Autodesk Fusion 360 part; units mm, degrees
(part 2 of 4)
  arc A294 (-148.6977, 144.525) -> (-148.6977, 141.525) centre (-148.6977, 143.025) ccw
  arc A295 (-138.6977, 141.525) -> (-138.6977, 144.525) centre (-138.6977, 143.025) ccw
  line L447 (-148.6977, 144.525) -> (-138.6977, 144.525)
  line L448 (-148.6977, 141.525) -> (-143.6977, 141.525)
  line L449 (-138.6977, 141.525) -> (-143.6977, 141.525)
  arc A296 (-128.6977, 144.525) -> (-128.6977, 141.525) centre (-128.6977, 143.025) ccw
  arc A297 (-118.6977, 141.525) -> (-118.6977, 144.525) centre (-118.6977, 143.025) ccw
  line L450 (-128.6977, 144.525) -> (-118.6977, 144.525)
  line L451 (-128.6977, 141.525) -> (-123.6977, 141.525)
  line L452 (-118.6977, 141.525) -> (-123.6977, 141.525)
  arc A298 (-228.6977, 154.525) -> (-228.6977, 151.525) centre (-228.6977, 153.025) ccw
  arc A299 (-218.6977, 151.525) -> (-218.6977, 154.525) centre (-218.6977, 153.025) ccw
  line L453 (-228.6977, 154.525) -> (-218.6977, 154.525)
  line L454 (-228.6977, 151.525) -> (-223.6977, 151.525)
  line L455 (-218.6977, 151.525) -> (-223.6977, 151.525)
  arc A300 (-208.6977, 154.525) -> (-208.6977, 151.525) centre (-208.6977, 153.025) ccw
  arc A301 (-198.6977, 151.525) -> (-198.6977, 154.525) centre (-198.6977, 153.025) ccw
  line L456 (-208.6977, 154.525) -> (-198.6977, 154.525)
  line L457 (-208.6977, 151.525) -> (-203.6977, 151.525)
  line L458 (-198.6977, 151.525) -> (-203.6977, 151.525)
  arc A302 (-188.6977, 154.525) -> (-188.6977, 151.525) centre (-188.6977, 153.025) ccw
  arc A303 (-178.6977, 151.525) -> (-178.6977, 154.525) centre (-178.6977, 153.025) ccw
  line L459 (-188.6977, 154.525) -> (-178.6977, 154.525)
  line L460 (-188.6977, 151.525) -> (-183.6977, 151.525)
  line L461 (-178.6977, 151.525) -> (-183.6977, 151.525)
  arc A304 (-168.6977, 154.525) -> (-168.6977, 151.525) centre (-168.6977, 153.025) ccw
  arc A305 (-158.6977, 151.525) -> (-158.6977, 154.525) centre (-158.6977, 153.025) ccw
  line L462 (-168.6977, 154.525) -> (-158.6977, 154.525)
  line L463 (-168.6977, 151.525) -> (-163.6977, 151.525)
  line L464 (-158.6977, 151.525) -> (-163.6977, 151.525)
  arc A306 (-148.6977, 154.525) -> (-148.6977, 151.525) centre (-148.6977, 153.025) ccw
  arc A307 (-138.6977, 151.525) -> (-138.6977, 154.525) centre (-138.6977, 153.025) ccw
  line L465 (-148.6977, 154.525) -> (-138.6977, 154.525)
  line L466 (-148.6977, 151.525) -> (-143.6977, 151.525)
  line L467 (-138.6977, 151.525) -> (-143.6977, 151.525)
  arc A308 (-128.6977, 154.525) -> (-128.6977, 151.525) centre (-128.6977, 153.025) ccw
  arc A309 (-118.6977, 151.525) -> (-118.6977, 154.525) centre (-118.6977, 153.025) ccw
  line L468 (-128.6977, 154.525) -> (-118.6977, 154.525)
  line L469 (-128.6977, 151.525) -> (-123.6977, 151.525)
  line L470 (-118.6977, 151.525) -> (-123.6977, 151.525)
  arc A310 (-228.6977, 164.525) -> (-228.6977, 161.525) centre (-228.6977, 163.025) ccw
  arc A311 (-218.6977, 161.525) -> (-218.6977, 164.525) centre (-218.6977, 163.025) ccw
  line L471 (-228.6977, 164.525) -> (-218.6977, 164.525)
  line L472 (-228.6977, 161.525) -> (-223.6977, 161.525)
  line L473 (-218.6977, 161.525) -> (-223.6977, 161.525)
  arc A312 (-208.6977, 164.525) -> (-208.6977, 161.525) centre (-208.6977, 163.025) ccw
  arc A313 (-198.6977, 161.525) -> (-198.6977, 164.525) centre (-198.6977, 163.025) ccw
  line L474 (-208.6977, 164.525) -> (-198.6977, 164.525)
  line L475 (-208.6977, 161.525) -> (-203.6977, 161.525)
  line L476 (-198.6977, 161.525) -> (-203.6977, 161.525)
  arc A314 (-188.6977, 164.525) -> (-188.6977, 161.525) centre (-188.6977, 163.025) ccw
  arc A315 (-178.6977, 161.525) -> (-178.6977, 164.525) centre (-178.6977, 163.025) ccw
  line L477 (-188.6977, 164.525) -> (-178.6977, 164.525)
  line L478 (-188.6977, 161.525) -> (-183.6977, 161.525)
  line L479 (-178.6977, 161.525) -> (-183.6977, 161.525)
  arc A316 (-168.6977, 164.525) -> (-168.6977, 161.525) centre (-168.6977, 163.025) ccw
  arc A317 (-158.6977, 161.525) -> (-158.6977, 164.525) centre (-158.6977, 163.025) ccw
  line L480 (-168.6977, 164.525) -> (-158.6977, 164.525)
  line L481 (-168.6977, 161.525) -> (-163.6977, 161.525)
  line L482 (-158.6977, 161.525) -> (-163.6977, 161.525)
  arc A318 (-148.6977, 164.525) -> (-148.6977, 161.525) centre (-148.6977, 163.025) ccw
  arc A319 (-138.6977, 161.525) -> (-138.6977, 164.525) centre (-138.6977, 163.025) ccw
  line L483 (-148.6977, 164.525) -> (-138.6977, 164.525)
  line L484 (-148.6977, 161.525) -> (-143.6977, 161.525)
  line L485 (-138.6977, 161.525) -> (-143.6977, 161.525)
  arc A320 (-208.6977, 174.525) -> (-208.6977, 171.525) centre (-208.6977, 173.025) ccw
  arc A321 (-198.6977, 171.525) -> (-198.6977, 174.525) centre (-198.6977, 173.025) ccw
  line L486 (-208.6977, 174.525) -> (-198.6977, 174.525)
  line L487 (-208.6977, 171.525) -> (-203.6977, 171.525)
  line L488 (-198.6977, 171.525) -> (-203.6977, 171.525)
  arc A322 (-188.6977, 174.525) -> (-188.6977, 171.525) centre (-188.6977, 173.025) ccw
  arc A323 (-178.6977, 171.525) -> (-178.6977, 174.525) centre (-178.6977, 173.025) ccw
  line L489 (-188.6977, 174.525) -> (-178.6977, 174.525)
  line L490 (-188.6977, 171.525) -> (-183.6977, 171.525)
  line L491 (-178.6977, 171.525) -> (-183.6977, 171.525)
  arc A324 (-168.6977, 174.525) -> (-168.6977, 171.525) centre (-168.6977, 173.025) ccw
  arc A325 (-158.6977, 171.525) -> (-158.6977, 174.525) centre (-158.6977, 173.025) ccw
  line L492 (-168.6977, 174.525) -> (-158.6977, 174.525)
  line L493 (-168.6977, 171.525) -> (-163.6977, 171.525)
  line L494 (-158.6977, 171.525) -> (-163.6977, 171.525)
  arc A326 (-148.6977, 174.525) -> (-148.6977, 171.525) centre (-148.6977, 173.025) ccw
  arc A327 (-138.6977, 171.525) -> (-138.6977, 174.525) centre (-138.6977, 173.025) ccw
  line L495 (-148.6977, 174.525) -> (-138.6977, 174.525)
  line L496 (-148.6977, 171.525) -> (-143.6977, 171.525)
  line L497 (-138.6977, 171.525) -> (-143.6977, 171.525)
  arc A328 (-208.6977, 184.525) -> (-208.6977, 181.525) centre (-208.6977, 183.025) ccw
  arc A329 (-198.6977, 181.525) -> (-198.6977, 184.525) centre (-198.6977, 183.025) ccw
  line L498 (-208.6977, 184.525) -> (-198.6977, 184.525)
  line L499 (-208.6977, 181.525) -> (-203.6977, 181.525)
  line L500 (-198.6977, 181.525) -> (-203.6977, 181.525)
  arc A330 (-188.6977, 184.525) -> (-188.6977, 181.525) centre (-188.6977, 183.025) ccw
  arc A331 (-178.6977, 181.525) -> (-178.6977, 184.525) centre (-178.6977, 183.025) ccw
  line L501 (-188.6977, 184.525) -> (-178.6977, 184.525)
  line L502 (-188.6977, 181.525) -> (-183.6977, 181.525)
  line L503 (-178.6977, 181.525) -> (-183.6977, 181.525)
  arc A332 (-168.6977, 184.525) -> (-168.6977, 181.525) centre (-168.6977, 183.025) ccw
  arc A333 (-158.6977, 181.525) -> (-158.6977, 184.525) centre (-158.6977, 183.025) ccw
  line L504 (-168.6977, 184.525) -> (-158.6977, 184.525)
  line L505 (-168.6977, 181.525) -> (-163.6977, 181.525)
  line L506 (-158.6977, 181.525) -> (-163.6977, 181.525)
  arc A334 (-148.6977, 184.525) -> (-148.6977, 181.525) centre (-148.6977, 183.025) ccw
  arc A335 (-138.6977, 181.525) -> (-138.6977, 184.525) centre (-138.6977, 183.025) ccw
  line L507 (-148.6977, 184.525) -> (-138.6977, 184.525)
  line L508 (-148.6977, 181.525) -> (-143.6977, 181.525)
  line L509 (-138.6977, 181.525) -> (-143.6977, 181.525)
  line L510 (-269.4662, 146.0492) -> (-250, 146.0218)
  line L511 (-269.5337, 0.009) -> (-249.9865, 0)
  line L512 (-105.9194, 0) -> (-90, 0)
  line L513 (-90, 0) -> (-60, 38.025)
  line L514 (-60, 38.025) -> (-17.3954, 46.901)
  line L515 (-17.3954, 99.149) -> (-17.3954, 46.901)
  line L516 (-60, 108.025) -> (-17.3954, 99.149)
  line L517 (-90, 146.05) -> (-60, 108.025)
  line L518 (-105.9194, 146.05) -> (-90, 146.05)
  line L519 (-269.4662, 146.0492) -> (-269.5337, 0.009)
  line L520 (-46.3999, 83.0262) -> (-53.3999, 83.0262)
  line L521 (-53.3999, 83.0262) -> (-53.3999, 63.0262)
  line L522 (-53.3999, 63.0262) -> (-46.3999, 63.0262)
  line L523 (-46.3999, 63.0262) -> (-46.3999, 83.0262)
  line L524 (-46.3999, 83.0262) -> (-53.3999, 63.0262) construction
  line L525 (-53.3999, 83.0262) -> (-46.3999, 63.0262) construction
  point P0 (-143.6977, 73.025)
  point P1 (-203.6977, -36.975)
  point P2 (-183.6977, -36.975)
  point P3 (-163.6977, -36.975)
  point P4 (-143.6977, -36.975)
  point P5 (-203.6977, -26.975)
  point P6 (-183.6977, -26.975)
  point P7 (-163.6977, -26.975)
  point P8 (-143.6977, -26.975)
  point P9 (-223.6977, -16.975)
  point P10 (-203.6977, -16.975)
  point P11 (-183.6977, -16.975)
  point P12 (-163.6977, -16.975)
  point P13 (-143.6977, -16.975)
  point P14 (-223.6977, -6.975)
  point P15 (-203.6977, -6.975)
  point P16 (-183.6977, -6.975)
  point P17 (-163.6977, -6.975)
  point P18 (-143.6977, -6.975)
  point P19 (-123.6977, -6.975)
  point P20 (-223.6977, 3.025)
  point P21 (-203.6977, 3.025)
  point P22 (-183.6977, 3.025)
  point P23 (-163.6977, 3.025)
  point P24 (-143.6977, 3.025)
  point P25 (-123.6977, 3.025)
  point P26 (-243.6977, 13.025)
  point P27 (-223.6977, 13.025)
  point P28 (-203.6977, 13.025)
  point P29 (-183.6977, 13.025)
  point P30 (-163.6977, 13.025)
  point P31 (-143.6977, 13.025)
  point P32 (-123.6977, 13.025)
  point P33 (-103.6977, 13.025)
  point P34 (-243.6977, 23.025)
  point P35 (-223.6977, 23.025)
  point P36 (-203.6977, 23.025)
  point P37 (-183.6977, 23.025)
  point P38 (-163.6977, 23.025)
  point P39 (-143.6977, 23.025)
  point P40 (-123.6977, 23.025)
  point P41 (-103.6977, 23.025)
  point P42 (-243.6977, 33.025)
  point P43 (-223.6977, 33.025)
  point P44 (-203.6977, 33.025)
  point P45 (-183.6977, 33.025)
  point P46 (-163.6977, 33.025)
  point P47 (-143.6977, 33.025)
  point P48 (-123.6977, 33.025)
  point P49 (-103.6977, 33.025)
  point P50 (-83.6977, 33.025)
  point P51 (-243.6977, 43.025)
  point P52 (-223.6977, 43.025)
  point P53 (-203.6977, 43.025)
  point P54 (-183.6977, 43.025)
  point P55 (-163.6977, 43.025)
  point P56 (-143.6977, 43.025)
  point P57 (-123.6977, 43.025)
  point P58 (-103.6977, 43.025)
  point P59 (-83.6977, 43.025)
  point P60 (-63.6977, 43.025)
  point P61 (-43.6977, 43.025)
  point P62 (-243.6977, 53.025)
  point P63 (-223.6977, 53.025)
  point P64 (-203.6977, 53.025)
  point P65 (-183.6977, 53.025)
  point P66 (-163.6977, 53.025)
  point P67 (-143.6977, 53.025)
  point P68 (-123.6977, 53.025)
  point P69 (-103.6977, 53.025)
  point P70 (-83.6977, 53.025)
  point P71 (-63.6977, 53.025)
  point P72 (-243.6977, 63.025)
  point P73 (-223.6977, 63.025)
  point P74 (-203.6977, 63.025)
  point P75 (-183.6977, 63.025)
  point P76 (-163.6977, 63.025)
  point P77 (-143.6977, 63.025)
  point P78 (-123.6977, 63.025)
  point P79 (-103.6977, 63.025)
  point P80 (-83.6977, 63.025)
  point P81 (-63.6977, 63.025)
  point P82 (-243.6977, 73.025)
  point P83 (-223.6977, 73.025)
  point P84 (-203.6977, 73.025)
  point P85 (-183.6977, 73.025)
  point P86 (-163.6977, 73.025)
  point P87 (-123.6977, 73.025)
  point P88 (-103.6977, 73.025)
  point P89 (-83.6977, 73.025)
  point P90 (-63.6977, 73.025)
  point P91 (-243.6977, 83.025)
  point P92 (-223.6977, 83.025)
  point P93 (-203.6977, 83.025)
  point P94 (-183.6977, 83.025)
  point P95 (-163.6977, 83.025)
  point P96 (-143.6977, 83.025)
  point P97 (-123.6977, 83.025)
  point P98 (-103.6977, 83.025)
  point P99 (-83.6977, 83.025)
  point P100 (-63.6977, 83.025)
  point P101 (-243.6977, 93.025)
  point P102 (-223.6977, 93.025)
  point P103 (-203.6977, 93.025)
  point P104 (-183.6977, 93.025)
  point P105 (-163.6977, 93.025)
  point P106 (-143.6977, 93.025)
  point P107 (-123.6977, 93.025)
  point P108 (-103.6977, 93.025)
  point P109 (-83.6977, 93.025)
  point P110 (-63.6977, 93.025)
  point P111 (-243.6977, 103.025)
  point P112 (-223.6977, 103.025)
  point P113 (-203.6977, 103.025)
  point P114 (-183.6977, 103.025)
  point P115 (-163.6977, 103.025)
  point P116 (-143.6977, 103.025)
  point P117 (-123.6977, 103.025)
  point P118 (-103.6977, 103.025)
  point P119 (-83.6977, 103.025)
  point P120 (-243.6977, 113.025)
  point P121 (-223.6977, 113.025)
  point P122 (-203.6977, 113.025)
  point P123 (-183.6977, 113.025)
  point P124 (-163.6977, 113.025)
  point P125 (-143.6977, 113.025)
  point P126 (-123.6977, 113.025)
  point P127 (-103.6977, 113.025)
  point P128 (-83.6977, 113.025)
  point P129 (-243.6977, 123.025)
  point P130 (-223.6977, 123.025)
  point P131 (-203.6977, 123.025)
  point P132 (-183.6977, 123.025)
  point P133 (-163.6977, 123.025)
  point P134 (-143.6977, 123.025)
  point P135 (-123.6977, 123.025)
  point P136 (-103.6977, 123.025)
  point P137 (-243.6977, 133.025)
  point P138 (-223.6977, 133.025)
  point P139 (-203.6977, 133.025)
  point P140 (-183.6977, 133.025)
  point P141 (-163.6977, 133.025)
  point P142 (-143.6977, 133.025)
  point P143 (-123.6977, 133.025)
  point P144 (-103.6977, 133.025)
  point P145 (-223.6977, 143.025)
  point P146 (-203.6977, 143.025)
  point P147 (-183.6977, 143.025)
  point P148 (-163.6977, 143.025)
  point P149 (-143.6977, 143.025)
  point P150 (-123.6977, 143.025)
  point P151 (-223.6977, 153.025)
  point P152 (-203.6977, 153.025)
  point P153 (-183.6977, 153.025)
  point P154 (-163.6977, 153.025)
  point P155 (-143.6977, 153.025)
  point P156 (-123.6977, 153.025)
  point P157 (-223.6977, 163.025)
  point P158 (-203.6977, 163.025)
  point P159 (-183.6977, 163.025)
  point P160 (-163.6977, 163.025)
  point P161 (-143.6977, 163.025)
  point P162 (-203.6977, 173.025)
  point P163 (-183.6977, 173.025)
  point P164 (-163.6977, 173.025)
  point P165 (-143.6977, 173.025)
  point P166 (-203.6977, 183.025)
  point P167 (-183.6977, 183.025)
  point P168 (-163.6977, 183.025)
  point P169 (-143.6977, 183.025)
  point P170 (-49.8999, 73.0262)
  dimension "d82" = 10
  dimension "d83" = 3
  dimension "d86" = 20
  dimension "d87" = 10
  dimension "d120" = 7
  dimension "d121" = 20
  dimension "d122" = 219.6
  constraint horizontal L6
  constraint parallel L6 L7
  constraint tangent A1 L8
  constraint horizontal L512
  constraint vertical L515
  constraint horizontal L518
  constraint perpendicular L511 L519
  constraint horizontal L520
  constraint perpendicular L520 L521
  constraint parallel L520 L522
  constraint parallel L521 L523
  constraint coincident L524 P170
  constraint coincident L525 P170
  measures "d82" distance of L7.start L7.end
  measures "d83" distance of A1.end L7.start
  measures "d120" distance of L521.end L522.end
  measures "d121" distance of L520.end L521.end
  measures "d122" distance of L519 P170
extrude "Extrude3" add sketch "Sketch2" along normal blind 5 makes body 1
sketch "Sketch8" plane through (0, 5, 0) normal (0, 1, 0) x (-1, 0, 0)
  arc A0 (248.6977, -94.525) -> (248.6977, -91.525) centre (248.6977, -93.025) ccw
  line L0 (248.6977, -94.525) -> (238.6977, -94.525)
  arc A1 (238.6977, -91.525) -> (238.6977, -94.525) centre (238.6977, -93.025) ccw
  line L1 (238.6977, -91.525) -> (248.6977, -91.525)
  arc A2 (208.6977, -154.525) -> (208.6977, -151.525) centre (208.6977, -153.025) ccw
  line L2 (208.6977, -154.525) -> (198.6977, -154.525)
  arc A3 (198.6977, -151.525) -> (198.6977, -154.525) centre (198.6977, -153.025) ccw
  line L3 (198.6977, -151.525) -> (208.6977, -151.525)
  arc A4 (168.6977, -64.525) -> (168.6977, -61.525) centre (168.6977, -63.025) ccw
  line L4 (168.6977, -64.525) -> (158.6977, -64.525)
  arc A5 (158.6977, -61.525) -> (158.6977, -64.525) centre (158.6977, -63.025) ccw
  line L5 (158.6977, -61.525) -> (168.6977, -61.525)
  arc A6 (228.6977, -114.525) -> (228.6977, -111.525) centre (228.6977, -113.025) ccw
  line L6 (228.6977, -114.525) -> (218.6977, -114.525)
  arc A7 (218.6977, -111.525) -> (218.6977, -114.525) centre (218.6977, -113.025) ccw
  line L7 (218.6977, -111.525) -> (228.6977, -111.525)
  arc A8 (128.6977, -154.525) -> (128.6977, -151.525) centre (128.6977, -153.025) ccw
  line L8 (128.6977, -154.525) -> (118.6977, -154.525)
  arc A9 (118.6977, -151.525) -> (118.6977, -154.525) centre (118.6977, -153.025) ccw
  line L9 (118.6977, -151.525) -> (128.6977, -151.525)
  arc A10 (228.6977, -144.525) -> (228.6977, -141.525) centre (228.6977, -143.025) ccw
  line L10 (228.6977, -144.525) -> (218.6977, -144.525)
  arc A11 (218.6977, -141.525) -> (218.6977, -144.525) centre (218.6977, -143.025) ccw
  line L11 (218.6977, -141.525) -> (228.6977, -141.525)
  arc A12 (168.6977, -144.525) -> (168.6977, -141.525) centre (168.6977, -143.025) ccw
  line L12 (168.6977, -144.525) -> (158.6977, -144.525)
  arc A13 (158.6977, -141.525) -> (158.6977, -144.525) centre (158.6977, -143.025) ccw
  line L13 (158.6977, -141.525) -> (168.6977, -141.525)
  arc A14 (168.6977, -154.525) -> (168.6977, -151.525) centre (168.6977, -153.025) ccw
  line L14 (168.6977, -154.525) -> (158.6977, -154.525)
  arc A15 (158.6977, -151.525) -> (158.6977, -154.525) centre (158.6977, -153.025) ccw
  line L15 (158.6977, -151.525) -> (168.6977, -151.525)
  arc A16 (248.6977, -74.525) -> (248.6977, -71.525) centre (248.6977, -73.025) ccw
  line L16 (248.6977, -74.525) -> (238.6977, -74.525)
  arc A17 (238.6977, -71.525) -> (238.6977, -74.525) centre (238.6977, -73.025) ccw
  line L17 (238.6977, -71.525) -> (248.6977, -71.525)
  arc A18 (248.6977, -114.525) -> (248.6977, -111.525) centre (248.6977, -113.025) ccw
  line L18 (248.6977, -114.525) -> (238.6977, -114.525)
  arc A19 (238.6977, -111.525) -> (238.6977, -114.525) centre (238.6977, -113.025) ccw
  line L19 (238.6977, -111.525) -> (248.6977, -111.525)
  arc A20 (148.6977, -174.525) -> (148.6977, -171.525) centre (148.6977, -173.025) ccw
  line L20 (148.6977, -174.525) -> (138.6977, -174.525)
  arc A21 (138.6977, -171.525) -> (138.6977, -174.525) centre (138.6977, -173.025) ccw
  line L21 (138.6977, -171.525) -> (148.6977, -171.525)
  arc A22 (128.6977, -134.525) -> (128.6977, -131.525) centre (128.6977, -133.025) ccw
  line L22 (128.6977, -134.525) -> (118.6977, -134.525)
  arc A23 (118.6977, -131.525) -> (118.6977, -134.525) centre (118.6977, -133.025) ccw
  line L23 (118.6977, -131.525) -> (128.6977, -131.525)
  arc A24 (128.6977, -144.525) -> (128.6977, -141.525) centre (128.6977, -143.025) ccw
  line L24 (128.6977, -144.525) -> (118.6977, -144.525)
  arc A25 (118.6977, -141.525) -> (118.6977, -144.525) centre (118.6977, -143.025) ccw
  line L25 (118.6977, -141.525) -> (128.6977, -141.525)
  arc A26 (88.6977, -84.525) -> (88.6977, -81.525) centre (88.6977, -83.025) ccw
  line L26 (88.6977, -84.525) -> (78.6977, -84.525)
  arc A27 (78.6977, -81.525) -> (78.6977, -84.525) centre (78.6977, -83.025) ccw
  line L27 (78.6977, -81.525) -> (88.6977, -81.525)
  arc A28 (228.6977, -74.525) -> (228.6977, -71.525) centre (228.6977, -73.025) ccw
  line L28 (228.6977, -74.525) -> (218.6977, -74.525)
  arc A29 (218.6977, -71.525) -> (218.6977, -74.525) centre (218.6977, -73.025) ccw
  line L29 (218.6977, -71.525) -> (228.6977, -71.525)
  arc A30 (108.6977, -104.525) -> (108.6977, -101.525) centre (108.6977, -103.025) ccw
  line L30 (108.6977, -104.525) -> (98.6977, -104.525)
  arc A31 (98.6977, -101.525) -> (98.6977, -104.525) centre (98.6977, -103.025) ccw
  line L31 (98.6977, -101.525) -> (108.6977, -101.525)
  arc A32 (108.6977, -134.525) -> (108.6977, -131.525) centre (108.6977, -133.025) ccw
  line L32 (108.6977, -134.525) -> (98.6977, -134.525)
  arc A33 (98.6977, -131.525) -> (98.6977, -134.525) centre (98.6977, -133.025) ccw
  line L33 (98.6977, -131.525) -> (108.6977, -131.525)
  arc A34 (148.6977, -134.525) -> (148.6977, -131.525) centre (148.6977, -133.025) ccw
  line L34 (148.6977, -134.525) -> (138.6977, -134.525)
  arc A35 (138.6977, -131.525) -> (138.6977, -134.525) centre (138.6977, -133.025) ccw
  line L35 (138.6977, -131.525) -> (148.6977, -131.525)
  arc A36 (168.6977, -184.525) -> (168.6977, -181.525) centre (168.6977, -183.025) ccw
  line L36 (168.6977, -184.525) -> (158.6977, -184.525)
  arc A37 (158.6977, -181.525) -> (158.6977, -184.525) centre (158.6977, -183.025) ccw
  line L37 (158.6977, -181.525) -> (168.6977, -181.525)
  arc A38 (148.6977, -114.525) -> (148.6977, -111.525) centre (148.6977, -113.025) ccw
  line L38 (148.6977, -114.525) -> (138.6977, -114.525)
  arc A39 (138.6977, -111.525) -> (138.6977, -114.525) centre (138.6977, -113.025) ccw
  line L39 (138.6977, -111.525) -> (148.6977, -111.525)
  arc A40 (228.6977, -104.525) -> (228.6977, -101.525) centre (228.6977, -103.025) ccw
  line L40 (228.6977, -104.525) -> (218.6977, -104.525)
  arc A41 (218.6977, -101.525) -> (218.6977, -104.525) centre (218.6977, -103.025) ccw
  line L41 (218.6977, -101.525) -> (228.6977, -101.525)
  arc A42 (68.6977, -74.525) -> (68.6977, -71.525) centre (68.6977, -73.025) ccw
  line L42 (68.6977, -74.525) -> (58.6977, -74.525)
  arc A43 (58.6977, -71.525) -> (58.6977, -74.525) centre (58.6977, -73.025) ccw
  line L43 (58.6977, -71.525) -> (68.6977, -71.525)
  arc A44 (188.6977, -64.525) -> (188.6977, -61.525) centre (188.6977, -63.025) ccw
  line L44 (188.6977, -64.525) -> (178.6977, -64.525)
  arc A45 (178.6977, -61.525) -> (178.6977, -64.525) centre (178.6977, -63.025) ccw
  line L45 (178.6977, -61.525) -> (188.6977, -61.525)
  arc A46 (188.6977, -104.525) -> (188.6977, -101.525) centre (188.6977, -103.025) ccw
  line L46 (188.6977, -104.525) -> (178.6977, -104.525)
  arc A47 (178.6977, -101.525) -> (178.6977, -104.525) centre (178.6977, -103.025) ccw
  line L47 (178.6977, -101.525) -> (188.6977, -101.525)
  arc A48 (248.6977, -134.525) -> (248.6977, -131.525) centre (248.6977, -133.025) ccw
  line L48 (248.6977, -134.525) -> (238.6977, -134.525)
  arc A49 (238.6977, -131.525) -> (238.6977, -134.525) centre (238.6977, -133.025) ccw
  line L49 (238.6977, -131.525) -> (248.6977, -131.525)
  arc A50 (128.6977, -64.525) -> (128.6977, -61.525) centre (128.6977, -63.025) ccw
  line L50 (128.6977, -64.525) -> (118.6977, -64.525)
  arc A51 (118.6977, -61.525) -> (118.6977, -64.525) centre (118.6977, -63.025) ccw
  line L51 (118.6977, -61.525) -> (128.6977, -61.525)
  arc A52 (88.6977, -114.525) -> (88.6977, -111.525) centre (88.6977, -113.025) ccw
  line L52 (88.6977, -114.525) -> (78.6977, -114.525)
  arc A53 (78.6977, -111.525) -> (78.6977, -114.525) centre (78.6977, -113.025) ccw
  line L53 (78.6977, -111.525) -> (88.6977, -111.525)
  arc A54 (108.6977, -74.525) -> (108.6977, -71.525) centre (108.6977, -73.025) ccw
  line L54 (108.6977, -74.525) -> (98.6977, -74.525)
  arc A55 (98.6977, -71.525) -> (98.6977, -74.525) centre (98.6977, -73.025) ccw
  line L55 (98.6977, -71.525) -> (108.6977, -71.525)
  arc A56 (188.6977, -154.525) -> (188.6977, -151.525) centre (188.6977, -153.025) ccw
  line L56 (188.6977, -154.525) -> (178.6977, -154.525)
  arc A57 (178.6977, -151.525) -> (178.6977, -154.525) centre (178.6977, -153.025) ccw
  line L57 (178.6977, -151.525) -> (188.6977, -151.525)
  arc A58 (228.6977, -124.525) -> (228.6977, -121.525) centre (228.6977, -123.025) ccw
  line L58 (228.6977, -124.525) -> (218.6977, -124.525)
  arc A59 (218.6977, -121.525) -> (218.6977, -124.525) centre (218.6977, -123.025) ccw
  line L59 (218.6977, -121.525) -> (228.6977, -121.525)
  arc A60 (148.6977, -164.525) -> (148.6977, -161.525) centre (148.6977, -163.025) ccw
  line L60 (148.6977, -164.525) -> (138.6977, -164.525)
  arc A61 (138.6977, -161.525) -> (138.6977, -164.525) centre (138.6977, -163.025) ccw
  line L61 (138.6977, -161.525) -> (148.6977, -161.525)
  arc A62 (248.6977, -84.525) -> (248.6977, -81.525) centre (248.6977, -83.025) ccw
  line L62 (248.6977, -84.525) -> (238.6977, -84.525)
  arc A63 (238.6977, -81.525) -> (238.6977, -84.525) centre (238.6977, -83.025) ccw
  line L63 (238.6977, -81.525) -> (248.6977, -81.525)
  arc A64 (88.6977, -94.525) -> (88.6977, -91.525) centre (88.6977, -93.025) ccw
  line L64 (88.6977, -94.525) -> (78.6977, -94.525)
  arc A65 (78.6977, -91.525) -> (78.6977, -94.525) centre (78.6977, -93.025) ccw
  line L65 (78.6977, -91.525) -> (88.6977, -91.525)
  arc A66 (68.6977, -84.525) -> (68.6977, -81.525) centre (68.6977, -83.025) ccw
  line L66 (68.6977, -84.525) -> (58.6977, -84.525)
  arc A67 (58.6977, -81.525) -> (58.6977, -84.525) centre (58.6977, -83.025) ccw
  line L67 (58.6977, -81.525) -> (68.6977, -81.525)
  arc A68 (188.6977, -74.525) -> (188.6977, -71.525) centre (188.6977, -73.025) ccw
  line L68 (188.6977, -74.525) -> (178.6977, -74.525)
  arc A69 (178.6977, -71.525) -> (178.6977, -74.525) centre (178.6977, -73.025) ccw
  line L69 (178.6977, -71.525) -> (188.6977, -71.525)
  arc A70 (148.6977, -94.525) -> (148.6977, -91.525) centre (148.6977, -93.025) ccw
  line L70 (148.6977, -94.525) -> (138.6977, -94.525)
  arc A71 (138.6977, -91.525) -> (138.6977, -94.525) centre (138.6977, -93.025) ccw
  line L71 (138.6977, -91.525) -> (148.6977, -91.525)
  arc A72 (168.6977, -134.525) -> (168.6977, -131.525) centre (168.6977, -133.025) ccw
  line L72 (168.6977, -134.525) -> (158.6977, -134.525)
  arc A73 (158.6977, -131.525) -> (158.6977, -134.525) centre (158.6977, -133.025) ccw
  line L73 (158.6977, -131.525) -> (168.6977, -131.525)
  arc A74 (108.6977, -124.525) -> (108.6977, -121.525) centre (108.6977, -123.025) ccw
  line L74 (108.6977, -124.525) -> (98.6977, -124.525)
  arc A75 (98.6977, -121.525) -> (98.6977, -124.525) centre (98.6977, -123.025) ccw
  line L75 (98.6977, -121.525) -> (108.6977, -121.525)
  arc A76 (208.6977, -184.525) -> (208.6977, -181.525) centre (208.6977, -183.025) ccw
  line L76 (208.6977, -184.525) -> (198.6977, -184.525)
  arc A77 (198.6977, -181.525) -> (198.6977, -184.525) centre (198.6977, -183.025) ccw
  line L77 (198.6977, -181.525) -> (208.6977, -181.525)
  arc A78 (208.6977, -64.525) -> (208.6977, -61.525) centre (208.6977, -63.025) ccw
  line L78 (208.6977, -64.525) -> (198.6977, -64.525)
  arc A79 (198.6977, -61.525) -> (198.6977, -64.525) centre (198.6977, -63.025) ccw
  line L79 (198.6977, -61.525) -> (208.6977, -61.525)
  arc A80 (168.6977, -114.525) -> (168.6977, -111.525) centre (168.6977, -113.025) ccw
  line L80 (168.6977, -114.525) -> (158.6977, -114.525)
  arc A81 (158.6977, -111.525) -> (158.6977, -114.525) centre (158.6977, -113.025) ccw
  line L81 (158.6977, -111.525) -> (168.6977, -111.525)
  arc A82 (228.6977, -94.525) -> (228.6977, -91.525) centre (228.6977, -93.025) ccw
  line L82 (228.6977, -94.525) -> (218.6977, -94.525)
  arc A83 (218.6977, -91.525) -> (218.6977, -94.525) centre (218.6977, -93.025) ccw
  line L83 (218.6977, -91.525) -> (228.6977, -91.525)
  arc A84 (168.6977, -164.525) -> (168.6977, -161.525) centre (168.6977, -163.025) ccw
  line L84 (168.6977, -164.525) -> (158.6977, -164.525)
  arc A85 (158.6977, -161.525) -> (158.6977, -164.525) centre (158.6977, -163.025) ccw
  line L85 (158.6977, -161.525) -> (168.6977, -161.525)
  arc A86 (108.6977, -94.525) -> (108.6977, -91.525) centre (108.6977, -93.025) ccw
  line L86 (108.6977, -94.525) -> (98.6977, -94.525)
  arc A87 (98.6977, -91.525) -> (98.6977, -94.525) centre (98.6977, -93.025) ccw
  line L87 (98.6977, -91.525) -> (108.6977, -91.525)
  arc A88 (208.6977, -134.525) -> (208.6977, -131.525) centre (208.6977, -133.025) ccw
  line L88 (208.6977, -134.525) -> (198.6977, -134.525)
  arc A89 (198.6977, -131.525) -> (198.6977, -134.525) centre (198.6977, -133.025) ccw
  line L89 (198.6977, -131.525) -> (208.6977, -131.525)
  arc A90 (208.6977, -164.525) -> (208.6977, -161.525) centre (208.6977, -163.025) ccw
  line L90 (208.6977, -164.525) -> (198.6977, -164.525)
  arc A91 (198.6977, -161.525) -> (198.6977, -164.525) centre (198.6977, -163.025) ccw
  line L91 (198.6977, -161.525) -> (208.6977, -161.525)
  arc A92 (128.6977, -84.525) -> (128.6977, -81.525) centre (128.6977, -83.025) ccw
  line L92 (128.6977, -84.525) -> (118.6977, -84.525)
  arc A93 (118.6977, -81.525) -> (118.6977, -84.525) centre (118.6977, -83.025) ccw
  line L93 (118.6977, -81.525) -> (128.6977, -81.525)
  arc A94 (128.6977, -104.525) -> (128.6977, -101.525) centre (128.6977, -103.025) ccw
  line L94 (128.6977, -104.525) -> (118.6977, -104.525)
  arc A95 (118.6977, -101.525) -> (118.6977, -104.525) centre (118.6977, -103.025) ccw
  line L95 (118.6977, -101.525) -> (128.6977, -101.525)
  arc A96 (208.6977, -74.525) -> (208.6977, -71.525) centre (208.6977, -73.025) ccw
  line L96 (208.6977, -74.525) -> (198.6977, -74.525)
  arc A97 (198.6977, -71.525) -> (198.6977, -74.525) centre (198.6977, -73.025) ccw
  line L97 (198.6977, -71.525) -> (208.6977, -71.525)
  arc A98 (228.6977, -84.525) -> (228.6977, -81.525) centre (228.6977, -83.025) ccw
  line L98 (228.6977, -84.525) -> (218.6977, -84.525)
  arc A99 (218.6977, -81.525) -> (218.6977, -84.525) centre (218.6977, -83.025) ccw
  line L99 (218.6977, -81.525) -> (228.6977, -81.525)
  arc A100 (188.6977, -114.525) -> (188.6977, -111.525) centre (188.6977, -113.025) ccw
  line L100 (188.6977, -114.525) -> (178.6977, -114.525)
  arc A101 (178.6977, -111.525) -> (178.6977, -114.525) centre (178.6977, -113.025) ccw
  line L101 (178.6977, -111.525) -> (188.6977, -111.525)
  arc A102 (88.6977, -104.525) -> (88.6977, -101.525) centre (88.6977, -103.025) ccw
  line L102 (88.6977, -104.525) -> (78.6977, -104.525)
  arc A103 (78.6977, -101.525) -> (78.6977, -104.525) centre (78.6977, -103.025) ccw
  line L103 (78.6977, -101.525) -> (88.6977, -101.525)
  arc A104 (168.6977, -74.525) -> (168.6977, -71.525) centre (168.6977, -73.025) ccw
  line L104 (168.6977, -74.525) -> (158.6977, -74.525)
  arc A105 (158.6977, -71.525) -> (158.6977, -74.525) centre (158.6977, -73.025) ccw
  line L105 (158.6977, -71.525) -> (168.6977, -71.525)
  arc A106 (148.6977, -184.525) -> (148.6977, -181.525) centre (148.6977, -183.025) ccw
  line L106 (148.6977, -184.525) -> (138.6977, -184.525)
  arc A107 (138.6977, -181.525) -> (138.6977, -184.525) centre (138.6977, -183.025) ccw
  line L107 (138.6977, -181.525) -> (148.6977, -181.525)
  arc A108 (248.6977, -104.525) -> (248.6977, -101.525) centre (248.6977, -103.025) ccw
  line L108 (248.6977, -104.525) -> (238.6977, -104.525)
  arc A109 (238.6977, -101.525) -> (238.6977, -104.525) centre (238.6977, -103.025) ccw
  line L109 (238.6977, -101.525) -> (248.6977, -101.525)
  arc A110 (108.6977, -114.525) -> (108.6977, -111.525) centre (108.6977, -113.025) ccw
  line L110 (108.6977, -114.525) -> (98.6977, -114.525)
  arc A111 (98.6977, -111.525) -> (98.6977, -114.525) centre (98.6977, -113.025) ccw
  line L111 (98.6977, -111.525) -> (108.6977, -111.525)
  arc A112 (188.6977, -134.525) -> (188.6977, -131.525) centre (188.6977, -133.025) ccw
  line L112 (188.6977, -134.525) -> (178.6977, -134.525)
  arc A113 (178.6977, -131.525) -> (178.6977, -134.525) centre (178.6977, -133.025) ccw
  line L113 (178.6977, -131.525) -> (188.6977, -131.525)
  arc A114 (208.6977, -84.525) -> (208.6977, -81.525) centre (208.6977, -83.025) ccw
  line L114 (208.6977, -84.525) -> (198.6977, -84.525)
  arc A115 (198.6977, -81.525) -> (198.6977, -84.525) centre (198.6977, -83.025) ccw
  line L115 (198.6977, -81.525) -> (208.6977, -81.525)
  arc A116 (208.6977, -114.525) -> (208.6977, -111.525) centre (208.6977, -113.025) ccw
  line L116 (208.6977, -114.525) -> (198.6977, -114.525)
  arc A117 (198.6977, -111.525) -> (198.6977, -114.525) centre (198.6977, -113.025) ccw
  line L117 (198.6977, -111.525) -> (208.6977, -111.525)
  arc A118 (208.6977, -94.525) -> (208.6977, -91.525) centre (208.6977, -93.025) ccw
  line L118 (208.6977, -94.525) -> (198.6977, -94.525)
  arc A119 (198.6977, -91.525) -> (198.6977, -94.525) centre (198.6977, -93.025) ccw
  line L119 (198.6977, -91.525) -> (208.6977, -91.525)
  arc A120 (68.6977, -94.525) -> (68.6977, -91.525) centre (68.6977, -93.025) ccw
  line L120 (68.6977, -94.525) -> (58.6977, -94.525)
  arc A121 (58.6977, -91.525) -> (58.6977, -94.525) centre (58.6977, -93.025) ccw
  line L121 (58.6977, -91.525) -> (68.6977, -91.525)
  arc A122 (88.6977, -74.525) -> (88.6977, -71.525) centre (88.6977, -73.025) ccw
  line L122 (88.6977, -74.525) -> (78.6977, -74.525)
  arc A123 (78.6977, -71.525) -> (78.6977, -74.525) centre (78.6977, -73.025) ccw
  line L123 (78.6977, -71.525) -> (88.6977, -71.525)
  arc A124 (188.6977, -84.525) -> (188.6977, -81.525) centre (188.6977, -83.025) ccw
  line L124 (188.6977, -84.525) -> (178.6977, -84.525)
  arc A125 (178.6977, -81.525) -> (178.6977, -84.525) centre (178.6977, -83.025) ccw
  line L125 (178.6977, -81.525) -> (188.6977, -81.525)
  arc A126 (128.6977, -74.525) -> (128.6977, -71.525) centre (128.6977, -73.025) ccw
  line L126 (128.6977, -74.525) -> (118.6977, -74.525)
  arc A127 (118.6977, -71.525) -> (118.6977, -74.525) centre (118.6977, -73.025) ccw
  line L127 (118.6977, -71.525) -> (128.6977, -71.525)
  arc A128 (108.6977, -64.525) -> (108.6977, -61.525) centre (108.6977, -63.025) ccw
  line L128 (108.6977, -64.525) -> (98.6977, -64.525)
  arc A129 (98.6977, -61.525) -> (98.6977, -64.525) centre (98.6977, -63.025) ccw
  line L129 (98.6977, -61.525) -> (108.6977, -61.525)
  arc A130 (208.6977, -144.525) -> (208.6977, -141.525) centre (208.6977, -143.025) ccw
  line L130 (208.6977, -144.525) -> (198.6977, -144.525)
  arc A131 (198.6977, -141.525) -> (198.6977, -144.525) centre (198.6977, -143.025) ccw
  line L131 (198.6977, -141.525) -> (208.6977, -141.525)
  arc A132 (128.6977, -124.525) -> (128.6977, -121.525) centre (128.6977, -123.025) ccw
  line L132 (128.6977, -124.525) -> (118.6977, -124.525)
  arc A133 (118.6977, -121.525) -> (118.6977, -124.525) centre (118.6977, -123.025) ccw
  line L133 (118.6977, -121.525) -> (128.6977, -121.525)
  arc A134 (148.6977, -64.525) -> (148.6977, -61.525) centre (148.6977, -63.025) ccw
  line L134 (148.6977, -64.525) -> (138.6977, -64.525)
  arc A135 (138.6977, -61.525) -> (138.6977, -64.525) centre (138.6977, -63.025) ccw
  line L135 (138.6977, -61.525) -> (148.6977, -61.525)
  arc A136 (148.6977, -124.525) -> (148.6977, -121.525) centre (148.6977, -123.025) ccw
  line L136 (148.6977, -124.525) -> (138.6977, -124.525)
  arc A137 (138.6977, -121.525) -> (138.6977, -124.525) centre (138.6977, -123.025) ccw
  line L137 (138.6977, -121.525) -> (148.6977, -121.525)
  arc A138 (188.6977, -164.525) -> (188.6977, -161.525) centre (188.6977, -163.025) ccw
  line L138 (188.6977, -164.525) -> (178.6977, -164.525)
  arc A139 (178.6977, -161.525) -> (178.6977, -164.525) centre (178.6977, -163.025) ccw
  line L139 (178.6977, -161.525) -> (188.6977, -161.525)
  arc A140 (208.6977, -174.525) -> (208.6977, -171.525) centre (208.6977, -173.025) ccw
  line L140 (208.6977, -174.525) -> (198.6977, -174.525)
  arc A141 (198.6977, -171.525) -> (198.6977, -174.525) centre (198.6977, -173.025) ccw
  line L141 (198.6977, -171.525) -> (208.6977, -171.525)
  arc A142 (188.6977, -184.525) -> (188.6977, -181.525) centre (188.6977, -183.025) ccw
  line L142 (188.6977, -184.525) -> (178.6977, -184.525)
  arc A143 (178.6977, -181.525) -> (178.6977, -184.525) centre (178.6977, -183.025) ccw
  line L143 (178.6977, -181.525) -> (188.6977, -181.525)
  arc A144 (228.6977, -134.525) -> (228.6977, -131.525) centre (228.6977, -133.025) ccw
  line L144 (228.6977, -134.525) -> (218.6977, -134.525)
  arc A145 (218.6977, -131.525) -> (218.6977, -134.525) centre (218.6977, -133.025) ccw
  line L145 (218.6977, -131.525) -> (228.6977, -131.525)
  arc A146 (188.6977, -124.525) -> (188.6977, -121.525) centre (188.6977, -123.025) ccw
  line L146 (188.6977, -124.525) -> (178.6977, -124.525)
  arc A147 (178.6977, -121.525) -> (178.6977, -124.525) centre (178.6977, -123.025) ccw
  line L147 (178.6977, -121.525) -> (188.6977, -121.525)
  arc A148 (68.6977, -64.525) -> (68.6977, -61.525) centre (68.6977, -63.025) ccw
  line L148 (68.6977, -64.525) -> (58.6977, -64.525)
  arc A149 (58.6977, -61.525) -> (58.6977, -64.525) centre (58.6977, -63.025) ccw
  line L149 (58.6977, -61.525) -> (68.6977, -61.525)
  arc A150 (188.6977, -144.525) -> (188.6977, -141.525) centre (188.6977, -143.025) ccw
  line L150 (188.6977, -144.525) -> (178.6977, -144.525)
  arc A151 (178.6977, -141.525) -> (178.6977, -144.525) centre (178.6977, -143.025) ccw
  line L151 (178.6977, -141.525) -> (188.6977, -141.525)
  arc A152 (228.6977, -164.525) -> (228.6977, -161.525) centre (228.6977, -163.025) ccw
  line L152 (228.6977, -164.525) -> (218.6977, -164.525)
  arc A153 (218.6977, -161.525) -> (218.6977, -164.525) centre (218.6977, -163.025) ccw
  line L153 (218.6977, -161.525) -> (228.6977, -161.525)
  arc A154 (148.6977, -84.525) -> (148.6977, -81.525) centre (148.6977, -83.025) ccw
  line L154 (148.6977, -84.525) -> (138.6977, -84.525)
  arc A155 (138.6977, -81.525) -> (138.6977, -84.525) centre (138.6977, -83.025) ccw
  line L155 (138.6977, -81.525) -> (148.6977, -81.525)
  arc A156 (168.6977, -124.525) -> (168.6977, -121.525) centre (168.6977, -123.025) ccw
  line L156 (168.6977, -124.525) -> (158.6977, -124.525)
  arc A157 (158.6977, -121.525) -> (158.6977, -124.525) centre (158.6977, -123.025) ccw
  line L157 (158.6977, -121.525) -> (168.6977, -121.525)
  arc A158 (148.6977, -144.525) -> (148.6977, -141.525) centre (148.6977, -143.025) ccw
  line L158 (148.6977, -144.525) -> (138.6977, -144.525)
  arc A159 (138.6977, -141.525) -> (138.6977, -144.525) centre (138.6977, -143.025) ccw
  line L159 (138.6977, -141.525) -> (148.6977, -141.525)
  arc A160 (168.6977, -84.525) -> (168.6977, -81.525) centre (168.6977, -83.025) ccw
  line L160 (168.6977, -84.525) -> (158.6977, -84.525)
  arc A161 (158.6977, -81.525) -> (158.6977, -84.525) centre (158.6977, -83.025) ccw
  line L161 (158.6977, -81.525) -> (168.6977, -81.525)
  arc A162 (168.6977, -94.525) -> (168.6977, -91.525) centre (168.6977, -93.025) ccw
  line L162 (168.6977, -94.525) -> (158.6977, -94.525)
  arc A163 (158.6977, -91.525) -> (158.6977, -94.525) centre (158.6977, -93.025) ccw
  line L163 (158.6977, -91.525) -> (168.6977, -91.525)
  arc A164 (148.6977, -104.525) -> (148.6977, -101.525) centre (148.6977, -103.025) ccw
  line L164 (148.6977, -104.525) -> (138.6977, -104.525)
  arc A165 (138.6977, -101.525) -> (138.6977, -104.525) centre (138.6977, -103.025) ccw
  line L165 (138.6977, -101.525) -> (148.6977, -101.525)
  arc A166 (128.6977, -114.525) -> (128.6977, -111.525) centre (128.6977, -113.025) ccw
  line L166 (128.6977, -114.525) -> (118.6977, -114.525)
  arc A167 (118.6977, -111.525) -> (118.6977, -114.525) centre (118.6977, -113.025) ccw
  line L167 (118.6977, -111.525) -> (128.6977, -111.525)
  arc A168 (228.6977, -154.525) -> (228.6977, -151.525) centre (228.6977, -153.025) ccw
  line L168 (228.6977, -154.525) -> (218.6977, -154.525)
  arc A169 (218.6977, -151.525) -> (218.6977, -154.525) centre (218.6977, -153.025) ccw
  line L169 (218.6977, -151.525) -> (228.6977, -151.525)
  arc A170 (128.6977, -94.525) -> (128.6977, -91.525) centre (128.6977, -93.025) ccw
  line L170 (128.6977, -94.525) -> (118.6977, -94.525)
  arc A171 (118.6977, -91.525) -> (118.6977, -94.525) centre (118.6977, -93.025) ccw
  line L171 (118.6977, -91.525) -> (128.6977, -91.525)
  arc A172 (88.6977, -64.525) -> (88.6977, -61.525) centre (88.6977, -63.025) ccw
  line L172 (88.6977, -64.525) -> (78.6977, -64.525)
  arc A173 (78.6977, -61.525) -> (78.6977, -64.525) centre (78.6977, -63.025) ccw
  line L173 (78.6977, -61.525) -> (88.6977, -61.525)
  arc A174 (108.6977, -84.525) -> (108.6977, -81.525) centre (108.6977, -83.025) ccw
  line L174 (108.6977, -84.525) -> (98.6977, -84.525)
  arc A175 (98.6977, -81.525) -> (98.6977, -84.525) centre (98.6977, -83.025) ccw
  line L175 (98.6977, -81.525) -> (108.6977, -81.525)
  arc A176 (208.6977, -124.525) -> (208.6977, -121.525) centre (208.6977, -123.025) ccw
  line L176 (208.6977, -124.525) -> (198.6977, -124.525)
  arc A177 (198.6977, -121.525) -> (198.6977, -124.525) centre (198.6977, -123.025) ccw
  line L177 (198.6977, -121.525) -> (208.6977, -121.525)
  arc A178 (168.6977, -104.525) -> (168.6977, -101.525) centre (168.6977, -103.025) ccw
  line L178 (168.6977, -104.525) -> (158.6977, -104.525)
  arc A179 (158.6977, -101.525) -> (158.6977, -104.525) centre (158.6977, -103.025) ccw
  line L179 (158.6977, -101.525) -> (168.6977, -101.525)
  arc A180 (188.6977, -174.525) -> (188.6977, -171.525) centre (188.6977, -173.025) ccw
  line L180 (188.6977, -174.525) -> (178.6977, -174.525)
  arc A181 (178.6977, -171.525) -> (178.6977, -174.525) centre (178.6977, -173.025) ccw
  line L181 (178.6977, -171.525) -> (188.6977, -171.525)
  arc A182 (168.6977, -174.525) -> (168.6977, -171.525) centre (168.6977, -173.025) ccw
  line L182 (168.6977, -174.525) -> (158.6977, -174.525)
  arc A183 (158.6977, -171.525) -> (158.6977, -174.525) centre (158.6977, -173.025) ccw
  line L183 (158.6977, -171.525) -> (168.6977, -171.525)
  arc A184 (248.6977, -124.525) -> (248.6977, -121.525) centre (248.6977, -123.025) ccw
  line L184 (248.6977, -124.525) -> (238.6977, -124.525)
  arc A185 (238.6977, -121.525) -> (238.6977, -124.525) centre (238.6977, -123.025) ccw
  line L185 (238.6977, -121.525) -> (248.6977, -121.525)
  arc A186 (148.6977, -154.525) -> (148.6977, -151.525) centre (148.6977, -153.025) ccw
  line L186 (148.6977, -154.525) -> (138.6977, -154.525)
  arc A187 (138.6977, -151.525) -> (138.6977, -154.525) centre (138.6977, -153.025) ccw
  line L187 (138.6977, -151.525) -> (148.6977, -151.525)
  arc A188 (188.6977, -94.525) -> (188.6977, -91.525) centre (188.6977, -93.025) ccw
  line L188 (188.6977, -94.525) -> (178.6977, -94.525)
  arc A189 (178.6977, -91.525) -> (178.6977, -94.525) centre (178.6977, -93.025) ccw
  line L189 (178.6977, -91.525) -> (188.6977, -91.525)
  arc A190 (208.6977, -104.525) -> (208.6977, -101.525) centre (208.6977, -103.025) ccw
  line L190 (208.6977, -104.525) -> (198.6977, -104.525)
  arc A191 (198.6977, -101.525) -> (198.6977, -104.525) centre (198.6977, -103.025) ccw
  line L191 (198.6977, -101.525) -> (208.6977, -101.525)
  arc A192 (208.6977, -14.525) -> (208.6977, -11.525) centre (208.6977, -13.025) ccw
  line L192 (208.6977, -14.525) -> (198.6977, -14.525)
  arc A193 (198.6977, -11.525) -> (198.6977, -14.525) centre (198.6977, -13.025) ccw
  line L193 (198.6977, -11.525) -> (208.6977, -11.525)
  arc A194 (248.6977, -14.525) -> (248.6977, -11.525) centre (248.6977, -13.025) ccw
  line L194 (248.6977, -14.525) -> (238.6977, -14.525)
  arc A195 (238.6977, -11.525) -> (238.6977, -14.525) centre (238.6977, -13.025) ccw
  line L195 (238.6977, -11.525) -> (248.6977, -11.525)
  arc A196 (128.6977, -4.525) -> (128.6977, -1.525) centre (128.6977, -3.025) ccw
  line L196 (128.6977, -4.525) -> (118.6977, -4.525)
  arc A197 (118.6977, -1.525) -> (118.6977, -4.525) centre (118.6977, -3.025) ccw
  line L197 (118.6977, -1.525) -> (128.6977, -1.525)
  arc A198 (228.6977, -14.525) -> (228.6977, -11.525) centre (228.6977, -13.025) ccw
  line L198 (228.6977, -14.525) -> (218.6977, -14.525)
  arc A199 (218.6977, -11.525) -> (218.6977, -14.525) centre (218.6977, -13.025) ccw
  line L199 (218.6977, -11.525) -> (228.6977, -11.525)
  arc A200 (148.6977, -74.525) -> (148.6977, -71.525) centre (148.6977, -73.025) ccw
  line L200 (148.6977, -74.525) -> (138.6977, -74.525)
  arc A201 (138.6977, -71.525) -> (138.6977, -74.525) centre (138.6977, -73.025) ccw
  line L201 (138.6977, -71.525) -> (148.6977, -71.525)
  arc A202 (248.6977, -24.525) -> (248.6977, -21.525) centre (248.6977, -23.025) ccw
  line L202 (248.6977, -24.525) -> (238.6977, -24.525)
  arc A203 (238.6977, -21.525) -> (238.6977, -24.525) centre (238.6977, -23.025) ccw
  line L203 (238.6977, -21.525) -> (248.6977, -21.525)
  arc A204 (188.6977, -44.525) -> (188.6977, -41.525) centre (188.6977, -43.025) ccw
  line L204 (188.6977, -44.525) -> (178.6977, -44.525)
  arc A205 (178.6977, -41.525) -> (178.6977, -44.525) centre (178.6977, -43.025) ccw
  line L205 (178.6977, -41.525) -> (188.6977, -41.525)
  arc A206 (128.6977, -34.525) -> (128.6977, -31.525) centre (128.6977, -33.025) ccw
  line L206 (128.6977, -34.525) -> (118.6977, -34.525)
  arc A207 (118.6977, -31.525) -> (118.6977, -34.525) centre (118.6977, -33.025) ccw
  line L207 (118.6977, -31.525) -> (128.6977, -31.525)
  arc A208 (228.6977, -24.525) -> (228.6977, -21.525) centre (228.6977, -23.025) ccw
  line L208 (228.6977, -24.525) -> (218.6977, -24.525)
  arc A209 (218.6977, -21.525) -> (218.6977, -24.525) centre (218.6977, -23.025) ccw
  line L209 (218.6977, -21.525) -> (228.6977, -21.525)
  arc A210 (148.6977, -54.525) -> (148.6977, -51.525) centre (148.6977, -53.025) ccw
  line L210 (148.6977, -54.525) -> (138.6977, -54.525)
  arc A211 (138.6977, -51.525) -> (138.6977, -54.525) centre (138.6977, -53.025) ccw
  line L211 (138.6977, -51.525) -> (148.6977, -51.525)
  arc A212 (208.6977, -44.525) -> (208.6977, -41.525) centre (208.6977, -43.025) ccw
  line L212 (208.6977, -44.525) -> (198.6977, -44.525)
  arc A213 (198.6977, -41.525) -> (198.6977, -44.525) centre (198.6977, -43.025) ccw
  line L213 (198.6977, -41.525) -> (208.6977, -41.525)
  arc A214 (208.6977, -24.525) -> (208.6977, -21.525) centre (208.6977, -23.025) ccw
  line L214 (208.6977, -24.525) -> (198.6977, -24.525)
  arc A215 (198.6977, -21.525) -> (198.6977, -24.525) centre (198.6977, -23.025) ccw
  line L215 (198.6977, -21.525) -> (208.6977, -21.525)
  arc A216 (88.6977, -54.525) -> (88.6977, -51.525) centre (88.6977, -53.025) ccw
  line L216 (88.6977, -54.525) -> (78.6977, -54.525)
  arc A217 (78.6977, -51.525) -> (78.6977, -54.525) centre (78.6977, -53.025) ccw
  line L217 (78.6977, -51.525) -> (88.6977, -51.525)
  arc A218 (68.6977, -54.525) -> (68.6977, -51.525) centre (68.6977, -53.025) ccw
  line L218 (68.6977, -54.525) -> (58.6977, -54.525)
  arc A219 (58.6977, -51.525) -> (58.6977, -54.525) centre (58.6977, -53.025) ccw
  line L219 (58.6977, -51.525) -> (68.6977, -51.525)
  arc A220 (248.6977, -44.525) -> (248.6977, -41.525) centre (248.6977, -43.025) ccw
  line L220 (248.6977, -44.525) -> (238.6977, -44.525)
  arc A221 (238.6977, -41.525) -> (238.6977, -44.525) centre (238.6977, -43.025) ccw
  line L221 (238.6977, -41.525) -> (248.6977, -41.525)
  arc A222 (108.6977, -14.525) -> (108.6977, -11.525) centre (108.6977, -13.025) ccw
  line L222 (108.6977, -14.525) -> (98.6977, -14.525)
  arc A223 (98.6977, -11.525) -> (98.6977, -14.525) centre (98.6977, -13.025) ccw
  line L223 (98.6977, -11.525) -> (108.6977, -11.525)
  arc A224 (248.6977, -64.525) -> (248.6977, -61.525) centre (248.6977, -63.025) ccw
  line L224 (248.6977, -64.525) -> (238.6977, -64.525)
  arc A225 (238.6977, -61.525) -> (238.6977, -64.525) centre (238.6977, -63.025) ccw
  line L225 (238.6977, -61.525) -> (248.6977, -61.525)
  arc A226 (208.6977, -34.525) -> (208.6977, -31.525) centre (208.6977, -33.025) ccw
  line L226 (208.6977, -34.525) -> (198.6977, -34.525)
  arc A227 (198.6977, -31.525) -> (198.6977, -34.525) centre (198.6977, -33.025) ccw
  line L227 (198.6977, -31.525) -> (208.6977, -31.525)
  arc A228 (188.6977, -54.525) -> (188.6977, -51.525) centre (188.6977, -53.025) ccw
  line L228 (188.6977, -54.525) -> (178.6977, -54.525)
  arc A229 (178.6977, -51.525) -> (178.6977, -54.525) centre (178.6977, -53.025) ccw
  line L229 (178.6977, -51.525) -> (188.6977, -51.525)
  arc A230 (128.6977, -54.525) -> (128.6977, -51.525) centre (128.6977, -53.025) ccw
  line L230 (128.6977, -54.525) -> (118.6977, -54.525)
  arc A231 (118.6977, -51.525) -> (118.6977, -54.525) centre (118.6977, -53.025) ccw
  line L231 (118.6977, -51.525) -> (128.6977, -51.525)
  arc A232 (168.6977, -14.525) -> (168.6977, -11.525) centre (168.6977, -13.025) ccw
  line L232 (168.6977, -14.525) -> (158.6977, -14.525)
  arc A233 (158.6977, -11.525) -> (158.6977, -14.525) centre (158.6977, -13.025) ccw
  line L233 (158.6977, -11.525) -> (168.6977, -11.525)
  arc A234 (228.6977, -44.525) -> (228.6977, -41.525) centre (228.6977, -43.025) ccw
  line L234 (228.6977, -44.525) -> (218.6977, -44.525)
  arc A235 (218.6977, -41.525) -> (218.6977, -44.525) centre (218.6977, -43.025) ccw
  line L235 (218.6977, -41.525) -> (228.6977, -41.525)
  arc A236 (228.6977, -54.525) -> (228.6977, -51.525) centre (228.6977, -53.025) ccw
  line L236 (228.6977, -54.525) -> (218.6977, -54.525)
  arc A237 (218.6977, -51.525) -> (218.6977, -54.525) centre (218.6977, -53.025) ccw
  line L237 (218.6977, -51.525) -> (228.6977, -51.525)
  arc A238 (168.6977, -24.525) -> (168.6977, -21.525) centre (168.6977, -23.025) ccw
  line L238 (168.6977, -24.525) -> (158.6977, -24.525)
  arc A239 (158.6977, -21.525) -> (158.6977, -24.525) centre (158.6977, -23.025) ccw
  line L239 (158.6977, -21.525) -> (168.6977, -21.525)
  arc A240 (188.6977, -14.525) -> (188.6977, -11.525) centre (188.6977, -13.025) ccw
  line L240 (188.6977, -14.525) -> (178.6977, -14.525)
  arc A241 (178.6977, -11.525) -> (178.6977, -14.525) centre (178.6977, -13.025) ccw
  line L241 (178.6977, -11.525) -> (188.6977, -11.525)
  arc A242 (168.6977, -34.525) -> (168.6977, -31.525) centre (168.6977, -33.025) ccw
  line L242 (168.6977, -34.525) -> (158.6977, -34.525)
  arc A243 (158.6977, -31.525) -> (158.6977, -34.525) centre (158.6977, -33.025) ccw
  line L243 (158.6977, -31.525) -> (168.6977, -31.525)
  arc A244 (128.6977, -44.525) -> (128.6977, -41.525) centre (128.6977, -43.025) ccw
  line L244 (128.6977, -44.525) -> (118.6977, -44.525)
  arc A245 (118.6977, -41.525) -> (118.6977, -44.525) centre (118.6977, -43.025) ccw
  line L245 (118.6977, -41.525) -> (128.6977, -41.525)
  arc A246 (88.6977, -44.525) -> (88.6977, -41.525) centre (88.6977, -43.025) ccw
  line L246 (88.6977, -44.525) -> (78.6977, -44.525)
  arc A247 (78.6977, -41.525) -> (78.6977, -44.525) centre (78.6977, -43.025) ccw
  line L247 (78.6977, -41.525) -> (88.6977, -41.525)
  arc A248 (248.6977, -34.525) -> (248.6977, -31.525) centre (248.6977, -33.025) ccw
  line L248 (248.6977, -34.525) -> (238.6977, -34.525)
  arc A249 (238.6977, -31.525) -> (238.6977, -34.525) centre (238.6977, -33.025) ccw
  line L249 (238.6977, -31.525) -> (248.6977, -31.525)
  arc A250 (188.6977, -24.525) -> (188.6977, -21.525) centre (188.6977, -23.025) ccw